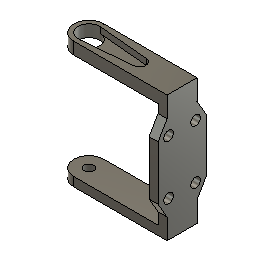
a-mu v12 (Autodesk Fusion 360 design; units mm, degrees)
Autodesk Fusion 360 part; units mm, degrees
note: some values were not read from the file. Set by a fixed rule: which sketch regions a step uses.
sketch "スケッチ1" plane through (0, 0, 0) normal (0, 1, 0) x (1, 0, 0)
  circle A0 centre (0, 0) radius 1.6
  circle A1 centre (0, 0) radius 5
  line L0 (0, 5) -> (30, 5)
  line L1 (30, 5) -> (30, -5)
  line L2 (30, -5) -> (0, -5)
  line L3 (0, -5) -> (0, 5)
  dimension "d1" = 3.2
  dimension "d2" = 30
  dimension "d3" = 10
  constraint coincident A0.centre A1.centre
  constraint concentric A0 A1
  constraint horizontal L0
  constraint vertical L1
  constraint horizontal L2
  constraint vertical L3
  constraint coincident A1 L0.start
  measures "d1" diameter of A0
  measures "d2" distance of L0.start L0.end
  measures "d3" distance of L0.start L2.end
extrude "押し出し1" add sketch "スケッチ1" along normal blind 3 contours A0 A1 L3 | A0 A1 L3 | A1 L0 L1 L2
sketch "スケッチ2" plane through (0, 3, 0) normal (0, 1, 0) x (-1, 0, 0)
  circle A0 centre (0, 0) radius 1.6
  arc A1 (0, -5) -> (0, 5) centre (0, 0) ccw
  line L0 (0, 5) -> (-30, 5)
  line L1 (-30, 5) -> (-30, -5)
  line L2 (-30, -5) -> (0, -5)
  line L3 (-30, -5) -> (-27, -5)
  line L4 (-27, -5) -> (-27, 5)
  line L5 (-27, 5) -> (-30, 5)
  line L6 (-30, 5) -> (-30, -5)
  dimension "d6" = 3
  dimension "d7" = 10
  constraint horizontal L3
  constraint vertical L4
  constraint horizontal L5
  constraint vertical L6
  constraint coincident L1.end L2.start
  measures "d6" distance of L1.end L3.end
  measures "d7" distance of L1.end L0.end
extrude "押し出し2" add sketch "スケッチ2" along normal blind 30 contours L0 L1 L2 L3 L4 L5 L6
sketch "スケッチ3" plane through (0, 33, 0) normal (0, 1, 0) x (-1, 0, 0)
  line L0 (-30, 5) -> (-30, -5)
  line L1 (-30, -5) -> (-27, -5)
  line L2 (-27, -5) -> (-27, 5)
  line L3 (-27, 5) -> (-30, 5)
  line L4 (-27, 5) -> (-27, -5)
  line L5 (-27, -5) -> (0, -5)
  arc A0 (0, -5) -> (0, 5) centre (0, 0) ccw
  line L6 (0, 5) -> (-27, 5)
  circle A1 centre (0, 0) radius 1.6
extrude "押し出し3" add sketch "スケッチ3" along normal blind 3
extrude "押し出し4" add 1 faces at (19.5096, 36, -0.1572) along direction (0, 1, 0) blind 3
extrude "押し出し5" cut 1 faces at (18.5333, 33, 0) along direction (0, 1, 0) blind 3
extrude "押し出し6" add 1 faces at (19.5096, 39, -0.1572) along direction (0, 1, 0) blind 2
extrude "押し出し7" cut 1 faces at (18.5333, 36, 0) along direction (0, 1, 0) blind 2
extrude "押し出し8" add 1 faces at (18.5333, 38, 0) along direction (0, -1, 0) blind 2
extrude "押し出し9" cut 1 faces at (19.5096, 41, -0.1572) along direction (0, -1, 0) blind 2
extrude "押し出し10" add 1 faces at (19.5096, 39, -0.1572) along direction (0, 1, 0) blind 1
sketch "スケッチ4" plane through (0, 40, 0) normal (0, 1, 0) x (-1, 0, 0)
  circle A0 centre (0, 0) radius 1.6
  line L0 (0, 5) -> (-30, 5)
  line L1 (-30, 5) -> (-30, -5)
  line L2 (-30, -5) -> (0, -5)
  arc A1 (0, -5) -> (0, 5) centre (0, 0) ccw
  circle A2 centre (0, 0) radius 3.6
  dimension "d26" = 7.2
  constraint coincident A0.centre A1.centre
  measures "d26" diameter of A2
extrude "押し出し11" cut sketch "スケッチ4" against normal blind 10 contours A2
sketch "スケッチ5" plane through (0, 40, 0) normal (0, 1, 0) x (-1, 0, 0)
  circle A0 centre (0, 0) radius 3.6
  line L0 (0, 5) -> (-30, 5)
  line L1 (-30, 5) -> (-30, -5)
  line L2 (-30, -5) -> (0, -5)
  arc A1 (0, -5) -> (0, 5) centre (0, 0) ccw
  circle A2 centre (0, 0) radius 3.6
  line L3 (0, 0) -> (-2.3505, 0)
  line L4 (-2.3505, 0) -> (-16.8505, 0)
  circle A3 centre (-16.8505, 0) radius 2.1
  line L5 (-17.0374, -2.0917) -> (-0.3205, -3.5857)
  line L6 (-17.0374, 2.0917) -> (-0.3205, 3.5857)
  dimension "d29" = 14.5
  dimension "d30" = 4.2
  constraint coincident A0.centre A1.centre
  constraint horizontal L3
  constraint parallel L3 L4
  constraint coincident L4.end A3.centre
  constraint coincident A3 L5.start
  constraint coincident A2 L5.end
  constraint tangent A2 L5
  constraint tangent A3 L5
  constraint coincident A3 L6.start
  constraint coincident A2 L6.end
  constraint tangent A2 L6
  constraint tangent A3 L6
  measures "d29" distance of L3.end L4.end
  measures "d30" diameter of A3
extrude "押し出し12" cut sketch "スケッチ5" against normal blind 2 contours A0 A2 L4 A3 L6 | A0 A2 L4 A3 L5 | A3
extrude "押し出し13" cut 1 faces at (18.5333, 3, 0) along direction (0, -1, 0) blind 2
extrude "押し出し14" add 1 faces at (20.5333, 0, 0) along direction (0, -1, 0) blind 2
sketch "スケッチ6" plane through (30, 0, 0) normal (1, 0, 0) x (0, 0, -1)
  line L0 (-5, 40) -> (-5, -2)
  line L1 (-5, -2) -> (5, -2)
  line L2 (5, -2) -> (5, 40)
  line L3 (5, 40) -> (-5, 40)
  line L4 (5, -2) -> (5, -1)
  line L5 (-5, 40) -> (5, -2)
  line L6 (12, 26.5) -> (-12, 26.5)
  line L7 (-12, 26.5) -> (-12, 11.5)
  line L8 (-12, 11.5) -> (12, 11.5)
  line L9 (12, 11.5) -> (12, 26.5)
  line L10 (12, 26.5) -> (-12, 11.5) construction
  line L11 (-12, 26.5) -> (12, 11.5) construction
  line L12 (-12, 26.5) -> (-9, 26.5)
  line L13 (-9, 26.5) -> (-9, 23.5)
  line L14 (-9, 23.5) -> (-12, 23.5)
  line L15 (-12, 23.5) -> (-12, 26.5)
  line L16 (-12, 11.5) -> (-9, 11.5)
  line L17 (-9, 11.5) -> (-9, 14.5)
  line L18 (-9, 14.5) -> (-12, 14.5)
  line L19 (-12, 14.5) -> (-12, 11.5)
  line L20 (12, 26.5) -> (9, 26.5)
  line L21 (9, 26.5) -> (9, 23.5)
  line L22 (9, 23.5) -> (12, 23.5)
  line L23 (12, 23.5) -> (12, 26.5)
  line L24 (12, 11.5) -> (9, 11.5)
  line L25 (9, 11.5) -> (9, 14.5)
  line L26 (9, 14.5) -> (12, 14.5)
  line L27 (12, 14.5) -> (12, 11.5)
  circle A0 centre (-9, 23.5) radius 1.6
  circle A1 centre (-9, 14.5) radius 1.6
  circle A2 centre (9, 14.5) radius 1.6
  circle A3 centre (9, 23.5) radius 1.6
  point P0 (0, 19)
  dimension "d37" = 24
  dimension "d38" = 15
  dimension "d39" = 3
  dimension "d40" = 3
  dimension "d41" = 3
  dimension "d42" = 3
  dimension "d43" = 3
  dimension "d44" = 3
  dimension "d45" = 3
  dimension "d46" = 3
  dimension "d47" = 3.2
  dimension "d48" = 3.2
  dimension "d49" = 3.2
  dimension "d50" = 3.2
  constraint coincident L1.end L2.start
  constraint coincident L2 L4.end
  constraint perpendicular L1 L4
  constraint coincident L0.start L3.end
  constraint perpendicular L6 L7
  constraint parallel L6 L8
  constraint parallel L7 L9
  constraint horizontal L6
  constraint coincident L10 P0
  constraint coincident L11 P0
  constraint midpoint L5 P0
  constraint horizontal L12
  constraint vertical L13
  constraint horizontal L14
  constraint vertical L15
  constraint horizontal L16
  constraint vertical L17
  constraint horizontal L18
  constraint vertical L19
  constraint horizontal L20
  constraint vertical L21
  constraint horizontal L22
  constraint vertical L23
  constraint horizontal L24
  constraint vertical L25
  constraint horizontal L26
  constraint vertical L27
  constraint coincident L13.end L14.start
  constraint coincident L17.end L18.start
  constraint coincident L25.end L26.start
  constraint coincident L21.end L22.start
  measures "d37" distance of L7.end L8.end
  measures "d38" distance of L6.end L7.end
  measures "d39" distance of L6.end L12.end
  measures "d40" distance of L6.end L14.end
  measures "d41" distance of L7.end L16.end
  measures "d42" distance of L7.end L18.end
  measures "d43" distance of L6.start L20.end
  measures "d44" distance of L6.start L22.end
  measures "d45" distance of L8.end L24.end
  measures "d46" distance of L8.end L26.end
  measures "d47" diameter of A0
  measures "d48" diameter of A1
  measures "d49" diameter of A2
  measures "d50" diameter of A3
extrude "押し出し15" add sketch "スケッチ6" against normal blind 3 contours L0 L6 L7 L8 L13 L14 L17 L18 A0 A1 | L6 L7 L12 L13 L14 L15 A0 | L2 L6 L8 L9 L21 L22 L25 L26 A2 A3 | L7 L8 L16 L17 L18 L19 A1 | L6 L9 L20 L21 L22 L23 A3 | L8 L9 L24 L25 L26 L27 A2
chamfer "面取り1" distance 2 angle 45 4 edges at (28.5, 11.5, -12) (28.5, 26.5, -12) (28.5, 26.5, 12) (28.5, 11.5, 12)
sketch "スケッチ7" plane through (30, 0, 0) normal (1, 0, 0) x (0, 0, -1)
  circle A0 centre (-9, 14.5) radius 1.6
  circle A1 centre (-9, 23.5) radius 1.6
  circle A2 centre (9, 23.5) radius 1.6
  circle A3 centre (9, 14.5) radius 1.6
  line L0 (-12, 13.5) -> (-10, 11.5)
  line L1 (-10, 11.5) -> (-5, 11.5)
  line L2 (-5, 11.5) -> (-5, -2)
  line L3 (-5, -2) -> (5, -2)
  line L4 (5, -2) -> (5, 11.5)
  line L5 (5, 11.5) -> (10, 11.5)
  line L6 (10, 11.5) -> (12, 13.5)
  line L7 (12, 13.5) -> (12, 24.5)
  line L8 (12, 24.5) -> (10, 26.5)
  line L9 (10, 26.5) -> (5, 26.5)
  line L10 (5, 26.5) -> (5, 40)
  line L11 (5, 40) -> (-5, 40)
  line L12 (-5, 40) -> (-5, 26.5)
  line L13 (-5, 26.5) -> (-10, 26.5)
  line L14 (-10, 26.5) -> (-12, 24.5)
  line L15 (-12, 24.5) -> (-12, 13.5)
  line L16 (-12, 19) -> (12, 19)
  line L17 (0, 19) -> (0, 15.95)
  line L18 (0, 15.95) -> (4, 15.95)
  line L19 (0, 15.95) -> (-4, 15.95)
  line L20 (-4, 15.95) -> (4, 15.95)
  line L21 (4, 15.95) -> (4, 10.95)
  line L22 (4, 10.95) -> (-4, 10.95)
  line L23 (-4, 10.95) -> (-4, 15.95)
  line L24 (-4, 15.95) -> (-4, 22.05)
  line L25 (-4, 22.05) -> (4, 22.05)
  line L26 (4, 22.05) -> (4, 27.05)
  line L27 (4, 27.05) -> (-4, 27.05)
  line L28 (-4, 27.05) -> (-4, 22.05)
  dimension "d54" = 3.05
  dimension "d55" = 4
  dimension "d56" = 4
  dimension "d57" = 8
  dimension "d58" = 5
  dimension "d59" = 6.1
  dimension "d60" = 8
  dimension "d61" = 5
  constraint midpoint L15 L16.start
  constraint midpoint L7 L16.end
  constraint midpoint L16 L17.start
  constraint perpendicular L16 L17
  constraint perpendicular L17 L18
  constraint perpendicular L17 L19
  constraint horizontal L20
  constraint vertical L21
  constraint horizontal L22
  constraint vertical L23
  constraint perpendicular L16 L24
  constraint horizontal L25
  constraint vertical L26
  constraint horizontal L27
  constraint vertical L28
  measures "d54" distance of L17.start L17.end
  measures "d55" distance of L17.end L18.end
  measures "d56" distance of L17.end L19.end
  measures "d57" distance of L19.end L18.end
  measures "d58" distance of L19.end L22.end
  measures "d59" distance of L19.end L24.end
  measures "d60" distance of L24.end L25.end
  measures "d61" distance of L24.end L27.end
extrude "押し出し16" cut sketch "スケッチ7" against normal blind 11 contours L18 L19 L20 L21 L22 L23 | L25 L26 L27 L28
chamfer "面取り2" distance 2 angle 45 4 edges at (28.5, 26.5, 5) (28.5, 26.5, -5) (28.5, 11.5, -5) (28.5, 11.5, 5)
extrude "押し出し17" cut 1 faces at (27, 4.5, -1.6667) along direction (1, 0, 0) blind 1
extrude "押し出し18" add 1 faces at (30, 3.5, -1.6667) along direction (1, 0, 0) blind 1
sketch "スケッチ8" plane through (31, 0, 0) normal (1, 0, 0) x (0, 0, -1)
  line L0 (4, 22.05) -> (-4, 22.05)
  line L1 (-4, 22.05) -> (-4, 27.05)
  line L2 (-4, 27.05) -> (4, 27.05)
  line L3 (4, 27.05) -> (4, 22.05)
  line L4 (4, 15.95) -> (4, 10.95)
  line L5 (4, 10.95) -> (-4, 10.95)
  line L6 (-4, 10.95) -> (-4, 15.95)
  line L7 (-4, 15.95) -> (4, 15.95)
  circle A0 centre (-9, 14.5) radius 1.6
  circle A1 centre (-9, 23.5) radius 1.6
  circle A2 centre (9, 23.5) radius 1.6
  circle A3 centre (9, 14.5) radius 1.6
  line L8 (-12, 13.5) -> (-10, 11.5)
  line L9 (-10, 11.5) -> (-7, 11.5)
  line L10 (-7, 11.5) -> (-5, 9.5)
  line L11 (-5, 9.5) -> (-5, -2)
  line L12 (-5, -2) -> (5, -2)
  line L13 (5, -2) -> (5, 9.5)
  line L14 (5, 9.5) -> (7, 11.5)
  line L15 (7, 11.5) -> (10, 11.5)
  line L16 (10, 11.5) -> (12, 13.5)
  line L17 (12, 13.5) -> (12, 24.5)
  line L18 (12, 24.5) -> (10, 26.5)
  line L19 (10, 26.5) -> (7, 26.5)
  line L20 (7, 26.5) -> (5, 28.5)
  line L21 (5, 28.5) -> (5, 40)
  line L22 (5, 40) -> (-5, 40)
  line L23 (-5, 40) -> (-5, 28.5)
  line L24 (-5, 28.5) -> (-7, 26.5)
  line L25 (-7, 26.5) -> (-10, 26.5)
  line L26 (-10, 26.5) -> (-12, 24.5)
  line L27 (-12, 24.5) -> (-12, 13.5)
  line L28 (-5, 28.5) -> (-5, 9.5)
  line L29 (5, 28.5) -> (5, 9.5)
  constraint coincident L23.end L24.start
  constraint coincident L10.end L11.start
  constraint coincident L20.end L21.start
  constraint coincident L13.end L14.start
extrude "押し出し19" cut sketch "スケッチ8" against normal blind 10 contours L8 L9 L10 L24 L25 L26 L27 L28 | L14 L15 L16 L17 L18 L19 L20 L29
sketch "スケッチ9" plane through (31, 0, 0) normal (1, 0, 0) x (0, 0, -1)
  line L0 (-5, 40) -> (-5, -2)
  line L1 (-5, -2) -> (5, -2)
  line L2 (5, -2) -> (5, 40)
  line L3 (5, 40) -> (-5, 40)
  line L4 (4, 22.05) -> (-4, 22.05)
  line L5 (-4, 22.05) -> (-4, 27.05)
  line L6 (-4, 27.05) -> (4, 27.05)
  line L7 (4, 27.05) -> (4, 22.05)
  line L8 (4, 15.95) -> (4, 10.95)
  line L9 (4, 10.95) -> (-4, 10.95)
  line L10 (-4, 10.95) -> (-4, 15.95)
  line L11 (-4, 15.95) -> (4, 15.95)
  line L12 (-4, 27.05) -> (4, 27.05)
  line L13 (4, 27.05) -> (4, 22.05)
  line L14 (4, 22.05) -> (-4, 22.05)
  line L15 (-4, 22.05) -> (-4, 27.05)
  line L16 (-4, 15.95) -> (4, 15.95)
  line L17 (4, 15.95) -> (4, 10.95)
  line L18 (4, 10.95) -> (-4, 10.95)
  line L19 (-4, 10.95) -> (-4, 15.95)
  constraint horizontal L12
  constraint vertical L13
  constraint horizontal L14
  constraint vertical L15
  constraint coincident L4.start L7.end
  constraint coincident L5.end L6.start
  constraint horizontal L16
  constraint vertical L17
  constraint horizontal L18
  constraint vertical L19
  constraint coincident L8.end L9.start
  constraint coincident L10.end L11.start
extrude "押し出し20" add sketch "スケッチ9" against normal blind 3 contours L4 L5 L6 L7 L12 L13 L14 L15 | L8 L9 L10 L11 L16 L17 L18 L19
sketch "スケッチ10" plane through (31, 0, 0) normal (1, 0, 0) x (0, 0, -1)
  line L0 (-5, 40) -> (-5, -2)
  line L1 (-5, -2) -> (5, -2)
  line L2 (5, -2) -> (5, 40)
  line L3 (5, 40) -> (-5, 40)
  line L4 (-5, 40) -> (5, -2)
  line L5 (4.5, 28) -> (-4.5, 28)
  line L6 (-4.5, 28) -> (-4.5, 10)
  line L7 (-4.5, 10) -> (4.5, 10)
  line L8 (4.5, 10) -> (4.5, 28)
  line L9 (4.5, 28) -> (-4.5, 10) construction
  line L10 (-4.5, 28) -> (4.5, 10) construction
  circle A0 centre (-4.5, 28) radius 1.6
  circle A1 centre (4.5, 28) radius 1.6
  circle A2 centre (-4.5, 10) radius 1.6
  circle A3 centre (4.5, 10) radius 1.6
  line L11 (-4.5, 28) -> (-7.3284, 30.8284)
  line L12 (-4.5, 28) -> (-0.5, 28) construction
  line L13 (-7.3284, 30.8284) -> (-5, 33.1569)
  line L14 (-4.5, 28) -> (-12, 28)
  line L15 (-7.3284, 30.8284) -> (-10.1569, 28)
  line L16 (-5, 33.1569) -> (-7.9773, 28)
  line L17 (-5, 33.1569) -> (0.9546, 33.1569) construction
  line L18 (-4.5, 10) -> (-11, 10)
  line L19 (-7.9773, 28) -> (-7.9773, 10)
  line L20 (-7.9773, 10) -> (-5, 4.8431)
  line L21 (-7.9773, 10) -> (-2.0227, 10) construction
  line L22 (4.5, 10) -> (11, 10)
  line L23 (0, 19) -> (0, 15)
  line L24 (5, 33.1569) -> (7.9773, 28)
  line L25 (7.9773, 28) -> (7.9773, 10)
  line L26 (7.9773, 10) -> (5, 4.8431)
  point P0 (0, 19)
  dimension "d73" = 9
  dimension "d74" = 18
  dimension "d75" = 3.2
  dimension "d76" = 3.2
  dimension "d77" = 3.2
  dimension "d78" = 3.2
  dimension "d79" = 135
  dimension "d80" = 4
  dimension "d81" = 120
  dimension "d82" = 60
  constraint coincident L0.start L3.end
  constraint coincident L1.end L2.start
  constraint perpendicular L5 L6
  constraint parallel L5 L7
  constraint parallel L6 L8
  constraint horizontal L5
  constraint coincident L9 P0
  constraint coincident L10 P0
  constraint midpoint L4 P0
  constraint coincident L5.end L6.start
  constraint coincident L5.start L8.end
  constraint coincident L6.end L7.start
  constraint coincident L7.end L8.start
  constraint horizontal L12
  constraint coincident L0 L13.end
  constraint perpendicular L11 L13
  constraint perpendicular L0 L14
  constraint coincident L14 L15.end
  constraint perpendicular L11 L15
  constraint horizontal L17
  constraint coincident L14 L16.end
  constraint perpendicular L6 L18
  constraint coincident L18 L19.end
  constraint perpendicular L18 L19
  constraint horizontal L21
  constraint coincident L0 L20.end
  constraint perpendicular L2 L22
  constraint coincident P0 L23.start
  constraint vertical L23
  constraint symmetric L13.end L23 L24.start
  constraint symmetric L16.end L23 L24.end
  constraint symmetric L19.end L23 L25.end
  constraint symmetric L20.end L23 L26.end
  measures "d73" distance of L6.end L7.end
  measures "d74" distance of L5.end L6.end
  measures "d75" diameter of A0
  measures "d76" diameter of A1
  measures "d77" diameter of A2
  measures "d78" diameter of A3
  measures "d79" angle of L11 L12
  measures "d80" distance of L5.end L11.end
  measures "d81" angle of L16 L17
  measures "d82" angle of L20 L21
extrude "押し出し21" add sketch "スケッチ10" against normal blind 3 contours L0 A0 L11 L16 | A0 L11 L14 L16 | L2 A1 A3 L22 L24 L25 | L0 A0 A2 L14 L18 L19 | L0 A2 L18 L20 | L2 A3 L22 L26
extrude "押し出し22" cut sketch "スケッチ10" against normal blind 3.5 contours L0 L5 A0 L11 | L2 L5 L8 A1 | L5 L8 A1 | L5 L6 A0 | L0 L11 L14 | L0 L6 A0 L14 | L0 L7 A2 L18 | L6 L7 A2 | L7 L8 A3 | L2 L7 A3 L22 | L2 L8 A3 L22 | L0 L6 A2 L18
